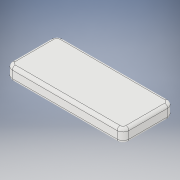
# Autodesk Inventor part: Mattress
Saved by Autodesk Inventor 2017 (Build 210142000, 142)
## iProperties
Created: 2016-10-24
Part Number: Mattress
Material: Generic
Document SubType Name: Modeling
Designer: andrew
Density: 1 g/cm^3
Appearance: White
Author: andrew
Autodesk Inventor part; units mm, degrees
ref_plane "YZ Plane" through (0, 0, 0) normal (1, 0, 0) x (0, 1, 0)
ref_plane "XZ Plane" through (0, 0, 0) normal (0, 1, 0) x (-1, 0, 0)
ref_plane "XY Plane" through (0, 0, 0) normal (0, 0, 1) x (1, 0, 0)
sketch "Sketch1" plane through (0, 0, 0) normal (0, 1, 0) x (-1, 0, 0)
  line L0 (-1003.3, 434.975) -> (1003.3, 434.975)
  line L1 (1003.3, 434.975) -> (1003.3, -434.975)
  line L2 (1003.3, -434.975) -> (-1003.3, -434.975)
  line L3 (-1003.3, -434.975) -> (-1003.3, 434.975)
  line L4 (-1003.3, 434.975) -> (1003.3, -434.975) construction
  line L5 (1003.3, 434.975) -> (-1003.3, -434.975) construction
  point P0 (0, 0)
  dimension "d0" = 869.95
  dimension "d3" = 2006.6
  constraints: 12 end point, 2 midpoint, 2 parallel, 1 horizontal, 1 perpendicular
  measures "d0" distance of L0.end L1.end
  measures "d3" distance of L0.start L0.end
extrude "Extrusion1" add sketch "Sketch1" along normal blind 228.6
fillet "Fillet1" radius 101.6 4 edges at (1003.3, 114.3, 434.975) (1003.3, 114.3, -434.975) (-1003.3, 114.3, 434.975) (-1003.3, 114.3, -434.975)
fillet "Fillet2" radius 50.8 16 edges at (973.542, 228.6, 405.217) (1003.3, 228.6, 0) (973.542, 228.6, -405.217) (0, 228.6, -434.975) (-973.542, 228.6, -405.217) (-1003.3, 228.6, 0) (-973.542, 228.6, 405.217) (0, 228.6, 434.975) (-973.542, 0, 405.217) (-1003.3, 0, 0) (-973.542, 0, -405.217) (0, 0, -434.975) (973.542, 0, -405.217) (1003.3, 0, 0) (973.542, 0, 405.217) (0, 0, 434.975)
body "Solid1"
